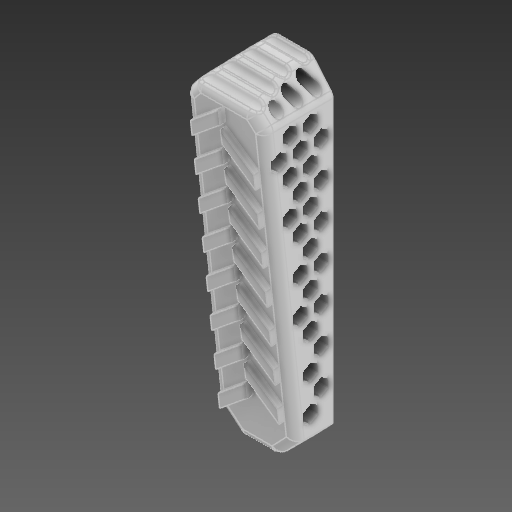
# Autodesk Inventor part: StockBack
Saved by Autodesk Inventor 2020.4 (Build 244396010, 396A)
## iProperties
Created: 2022-09-17
Part Number: StockBack
Material: Generic
Document SubType Name: Modeling
Designer: Val
Density: 1 g/cm^3
Appearance: Default
Author: Val
Autodesk Inventor part; units mm, degrees
ref_plane "Work Plane1" through (-11.1125, 103.225, 25.0771) normal (0, 0, -1) x (-1, 0, 0)
ref_plane "Work Plane2" through (-8.3683, 113.0409, 21.1281) normal (0, -0.1094954, 0.9939873) x (1, 0, 0)
ref_plane "YZ Plane" through (0, 0, 0) normal (1, 0, 0) x (0, 1, 0)
sketch "Base" plane through (0, 0, 0) normal (0, 0, 1) x (1, 0, 0)
  line L0 (0, 119.9075) -> (0, 0) construction
  line L1 (6.6224, 0) -> (0, 0)
  line L2 (14.2875, 7.9536) -> (6.6224, 0)
  line L3 (14.2875, 110.8887) -> (14.2875, 7.9536)
  line L4 (6.6224, 119.9075) -> (14.2875, 110.8887)
  line L5 (0, 119.9075) -> (6.6224, 119.9075)
  line L6 (0, 119.9075) -> (0, 0) construction
  line L7 (0, 119.9075) -> (-6.6224, 119.9075)
  line L8 (-6.6224, 119.9075) -> (-14.2875, 110.8887)
  line L9 (-14.2875, 110.8887) -> (-14.2875, 7.9536)
  line L10 (-14.2875, 7.9536) -> (-6.6224, 0)
  line L11 (-6.6224, 0) -> (0, 0)
  dimension "d0" = 136.058
  dimension "d1" = 139.638
  dimension "d2" = 90
  dimension "d3" = 40.362
  dimension "d4" = 90
  dimension "d5" = 43.942
  dimension "d6" = 14.2875
  dimension "d7" = 28.575
  dimension "d8" = 119.9075
  dimension "d9" = 14.2875
  dimension "d10" = 4.7684
  dimension "d11" = 82.6993
  dimension "d12" = 0
  dimension "d13" = 82.6993
  dimension "d14" = 4.7684
  constraints: 24 end point, 3 parallel, 1 horizontal, 1 vertical
  measures "d0" angle of L2 L3
  measures "d1" angle of L3 L4
  measures "d2" angle of L3 L7
  measures "d3" angle of L3 L8
  measures "d4" angle of L3 L11
  measures "d5" angle of L3 L10
  measures "d6" distance between parallel lines of L0 L3
  measures "d7" distance between parallel lines of L3 L9
  measures "d8" distance between parallel lines of L1 L5
  measures "d9" distance from line of point (0, 0) L3
  measures "d10" distance from line of point (0, 0) L2
  measures "d11" distance from line of point (0, 0) L4
  measures "d12" distance from line of point (0, 0) L1
  measures "d13" distance from line of point (0, 0) L8
  measures "d14" distance from line of point (0, 0) L10
extrude "BaseFeature" add sketch "Base" along normal blind 25.4
sketch "StockShapeProfile" plane through (-14.2875, 7.9536, 0) normal (-1, 0, 0) x (0, 0, 1)
  line L0 (-123.6771, 148.6169) -> (-186.3503, 165.9719) projected
  line L1 (-123.6771, 148.6169) -> (25.4, 107.3356)
  line L2 (-123.6771, 148.6169) -> (25.4, 148.6169)
  line L3 (25.4, 107.3356) -> (25.4, 148.6169)
  line L4 (25.4, 102.9352) -> (25.4, 0) projected
  point P0 (0, -7.9536)
  constraints: 6 end point, 2 collinear, 1 horizontal, 1 perpendicular
extrude "StockShapeFeature" cut sketch "StockShapeProfile" against normal through all both and the other way through all
sketch "StockProfile" plane through (-14.2875, 7.9536, 0) normal (-1, 0, 0) x (0, 0, 1)
  line L0 (25.4, 107.3356) -> (25.4, 102.9352) projected
  line L1 (25.4, 107.3356) -> (12.7, -7.9536)
  line L2 (0, -7.9536) -> (25.4, -7.9536) projected
  line L3 (25.4, 0) -> (25.4, -7.9536) projected
  line L4 (12.7, -7.9536) -> (25.4, -7.9536)
  line L5 (25.4, -7.9536) -> (25.4, 107.3356)
  constraints: 6 end point, 1 horizontal, 1 midpoint, 1 perpendicular
extrude "StockProfieFeature" cut sketch "StockProfile" against normal through all
fillet "StockFilletsFeature" radius 3.175 18 edges at (-14.2875, 110.8887, 12.4576) (-8.5849, 117.5983, 17.0611) (8.5849, 117.5983, 17.0611) (-14.2875, 7.9536, 6.7881) (-14.2875, 59.4212, 19.2457) (-12.4175, 113.089, 25.1576) (0, 115.2892, 25.4) (-10.4549, 3.9768, 13.1381) (10.4549, 3.9768, 13.1381) (14.2875, 59.4212, 19.2457) (14.2875, 110.8887, 12.4576) (12.4175, 113.089, 25.1576) (-6.6224, 119.9075, 4.3611) (6.6224, 119.9075, 4.3611) (3.3112, 119.9075, 8.7222) (-6.6224, 0, 6.35) (6.6224, 0, 6.35) (3.3112, 0, 12.7)
sketch "StockHoneycomb" plane through (-14.2875, 7.9536, 0) normal (-1, 0, 0) x (0, 0, 1)
  line L0 (7.9734, 94.5852) -> (5.2237, 96.1727)
  line L1 (5.2237, 96.1727) -> (5.2237, 99.3477)
  line L2 (5.2237, 99.3477) -> (7.9734, 100.9352)
  line L3 (7.9734, 100.9352) -> (10.723, 99.3477)
  line L4 (10.723, 99.3477) -> (10.723, 96.1727)
  line L5 (10.723, 96.1727) -> (7.9734, 94.5852)
  line L6 (0, 102.9352) -> (24.9153, 102.9352) projected
  line L7 (14.4726, 92.8531) -> (14.4726, 89.6781)
  line L8 (14.4726, 89.6781) -> (11.723, 88.0906)
  line L9 (11.723, 88.0906) -> (8.9734, 89.6781)
  line L10 (8.9734, 89.6781) -> (8.9734, 92.8531)
  line L11 (8.9734, 92.8531) -> (11.723, 94.4406)
  line L12 (11.723, 94.4406) -> (14.4726, 92.8531)
  line L13 (18.2222, 99.3477) -> (18.2222, 96.1727)
  line L14 (18.2222, 96.1727) -> (15.4726, 94.5852)
  line L15 (15.4726, 94.5852) -> (12.723, 96.1727)
  line L16 (12.723, 96.1727) -> (12.723, 99.3477)
  line L17 (12.723, 99.3477) -> (15.4726, 100.9352)
  line L18 (15.4726, 100.9352) -> (18.2222, 99.3477)
  line L19 (19.2222, 94.4406) -> (21.9719, 92.8531)
  line L20 (21.9719, 92.8531) -> (21.9719, 89.6781)
  line L21 (21.9719, 89.6781) -> (19.2222, 88.0906)
  line L22 (19.2222, 88.0906) -> (16.4726, 89.6781)
  line L23 (16.4726, 89.6781) -> (16.4726, 92.8531)
  line L24 (16.4726, 92.8531) -> (19.2222, 94.4406)
  line L25 (6.9734, 92.8531) -> (6.9734, 89.6781)
  line L26 (6.9734, 89.6781) -> (4.2237, 88.0906)
  line L27 (4.2237, 88.0906) -> (1.4741, 89.6781)
  line L28 (1.4741, 89.6781) -> (1.4741, 92.8531)
  line L29 (1.4741, 92.8531) -> (4.2237, 94.4406)
  line L30 (4.2237, 94.4406) -> (6.9734, 92.8531)
  line L31 (13.5761, 0) -> (24.9153, 102.9352) projected
  line L32 (10.723, 99.3477) -> (12.723, 99.3477) construction
  line L33 (4.2237, 91.2656) -> (19.2222, 91.2656) construction
  line L34 (7.9734, 87.9461) -> (5.2237, 86.3586)
  line L35 (5.2237, 86.3586) -> (5.2237, 83.1836)
  line L36 (5.2237, 83.1836) -> (7.9734, 81.5961)
  line L37 (7.9734, 81.5961) -> (10.723, 83.1836)
  line L38 (10.723, 83.1836) -> (10.723, 86.3586)
  line L39 (10.723, 86.3586) -> (7.9734, 87.9461)
  line L40 (18.2222, 83.1836) -> (18.2222, 86.3586)
  line L41 (18.2222, 86.3586) -> (15.4726, 87.9461)
  line L42 (15.4726, 87.9461) -> (12.723, 86.3586)
  line L43 (12.723, 86.3586) -> (12.723, 83.1836)
  line L44 (12.723, 83.1836) -> (15.4726, 81.5961)
  line L45 (15.4726, 81.5961) -> (18.2222, 83.1836)
  line L46 (5.2237, 84.7711) -> (18.2222, 84.7711) construction
  line L47 (14.4726, 76.689) -> (14.4726, 79.864)
  line L48 (14.4726, 79.864) -> (11.723, 81.4515)
  line L49 (11.723, 81.4515) -> (8.9734, 79.864)
  line L50 (8.9734, 79.864) -> (8.9734, 76.689)
  line L51 (8.9734, 76.689) -> (11.723, 75.1015)
  line L52 (11.723, 75.1015) -> (14.4726, 76.689)
  line L53 (19.2222, 75.1015) -> (21.9719, 76.689) construction
  line L54 (21.9719, 76.689) -> (21.9719, 79.864) construction
  line L55 (21.9719, 79.864) -> (19.2222, 81.4515) construction
  line L56 (19.2222, 81.4515) -> (16.4726, 79.864) construction
  line L57 (16.4726, 79.864) -> (16.4726, 76.689) construction
  line L58 (16.4726, 76.689) -> (19.2222, 75.1015) construction
  line L59 (6.9734, 76.689) -> (6.9734, 79.864)
  line L60 (6.9734, 79.864) -> (4.2237, 81.4515)
  line L61 (4.2237, 81.4515) -> (1.4741, 79.864)
  line L62 (1.4741, 79.864) -> (1.4741, 76.689)
  line L63 (1.4741, 76.689) -> (4.2237, 75.1015)
  line L64 (4.2237, 75.1015) -> (6.9734, 76.689)
  line L65 (4.2237, 78.2765) -> (19.2222, 78.2765) construction
  line L66 (5.2237, 70.1945) -> (5.2237, 73.3695)
  line L67 (5.2237, 73.3695) -> (7.9734, 74.957)
  line L68 (7.9734, 68.607) -> (5.2237, 70.1945)
  line L69 (10.723, 70.1945) -> (7.9734, 68.607)
  line L70 (10.723, 73.3695) -> (10.723, 70.1945)
  line L71 (7.9734, 74.957) -> (10.723, 73.3695)
  line L72 (12.723, 73.3695) -> (15.4726, 74.957)
  line L73 (15.4726, 74.957) -> (18.2222, 73.3695)
  line L74 (12.723, 70.1945) -> (12.723, 73.3695)
  line L75 (15.4726, 68.607) -> (12.723, 70.1945)
  line L76 (18.2222, 70.1945) -> (15.4726, 68.607)
  line L77 (18.2222, 73.3695) -> (18.2222, 70.1945)
  line L78 (0, 111.9539) -> (8.7222, 111.9539) construction
  line L79 (4.1309, 105.8244) -> (5.8691, 108.835) construction
  line L80 (5.8629, 104.8244) -> (7.6012, 107.835)
  line L81 (4.1371, 109.835) -> (2.3988, 106.8244)
  arc A0 (2.3988, 106.8244) -> (5.8629, 104.8244) centre (4.1309, 105.8244) ccw
  arc A1 (7.6012, 107.835) -> (4.1371, 109.835) centre (5.8691, 108.835) ccw
  line L82 (11.0591, 105.8244) -> (12.1387, 107.6942) construction
  line L83 (9.327, 106.8244) -> (10.4066, 108.6942)
  line L84 (13.8707, 106.6942) -> (12.7911, 104.8244)
  arc A2 (9.327, 106.8244) -> (12.7911, 104.8244) centre (11.0591, 105.8244) ccw
  arc A3 (13.8707, 106.6942) -> (10.4066, 108.6942) centre (12.1387, 107.6942) ccw
  line L85 (11.723, 68.4624) -> (14.4726, 66.8749)
  line L86 (14.4726, 66.8749) -> (14.4726, 63.6999)
  line L87 (14.4726, 63.6999) -> (11.723, 62.1124)
  line L88 (11.723, 62.1124) -> (8.9734, 63.6999)
  line L89 (8.9734, 63.6999) -> (8.9734, 66.8749)
  line L90 (8.9734, 66.8749) -> (11.723, 68.4624)
  line L91 (4.2237, 68.4624) -> (6.9734, 66.8749)
  line L92 (6.9734, 66.8749) -> (6.9734, 63.6999)
  line L93 (6.9734, 63.6999) -> (4.2237, 62.1124)
  line L94 (4.2237, 62.1124) -> (1.4741, 63.6999)
  line L95 (1.4741, 63.6999) -> (1.4741, 66.8749)
  line L96 (1.4741, 66.8749) -> (4.2237, 68.4624)
  line L97 (7.9734, 61.9679) -> (10.723, 60.3804)
  line L98 (10.723, 60.3804) -> (10.723, 57.2054)
  line L99 (10.723, 57.2054) -> (7.9734, 55.6179)
  line L100 (7.9734, 55.6179) -> (5.2237, 57.2054)
  line L101 (5.2237, 57.2054) -> (5.2237, 60.3804)
  line L102 (5.2237, 60.3804) -> (7.9734, 61.9679)
  line L103 (0, 110.835) -> (8.2907, 110.835) projected
  line L104 (21.5925, 103.8244) -> (0, 103.8244) projected
  line L105 (8.2907, 110.835) -> (21.9482, 107.0531) projected
  line L106 (0, 110.835) -> (0, 103.8244) projected
  line L107 (17.9873, 105.8244) -> (18.1119, 106.0402) construction
  line L108 (19.7193, 104.8244) -> (19.8439, 105.0402)
  line L109 (16.3798, 107.0402) -> (16.2552, 106.8244)
  arc A4 (16.2552, 106.8244) -> (19.7193, 104.8244) centre (17.9873, 105.8244) ccw
  arc A5 (19.8439, 105.0402) -> (16.3798, 107.0402) centre (18.1119, 106.0402) ccw
  point P0 (0, -7.9536)
  point P1 (7.9734, 97.7602)
  point P2 (11.723, 91.2656)
  point P3 (15.4726, 97.7602)
  point P4 (18.2222, 71.782)
  point P5 (5, 107.3297)
  point P6 (11.5989, 106.7593)
  point P7 (11.723, 65.2874)
  point P8 (4.2237, 65.2874)
  point P9 (7.9734, 58.7929)
  point P10 (18.0496, 105.9323)
  dimension "d21" = 3.175
  dimension "d22" = 2
  dimension "d24" = 2
  dimension "d25" = 2
  dimension "d26" = 2
  dimension "d27" = 2
  dimension "d28" = 2
  dimension "d29" = 2
  dimension "d30" = 2
  dimension "d31" = 1.4741
  dimension "d44" = 2
  dimension "d45" = 2
  dimension "d46" = 2
  dimension "d47" = 2
  dimension "d48" = 2
  dimension "d49" = 2
  dimension "d69" = 60
  dimension "d70" = 2
  dimension "d71" = 2
  dimension "d72" = 5
  dimension "d73" = 2
  constraints: 212 end point, 45 symmetric about line, 18 parallel, 18 tangent, 12 point on circle, 6 centre point, 5 midpoint, 2 equal radius, 1 horizontal, 104 other
  measures "d21" distance of L1.end L2.end
  measures "d22" distance from line of L6 L2.end
  measures "d24" distance between parallel lines of L5 L11
  measures "d25" distance between parallel lines of L15 L12
  measures "d26" distance between parallel lines of L4 L16
  measures "d27" distance between parallel lines of L24 L14
  measures "d28" distance between parallel lines of L30 L0
  measures "d29" distance between parallel lines of L10 L25
  measures "d30" distance between parallel lines of L23 L7
  measures "d31" distance from line of L31 L20.end
  measures "d44" distance from line of L75 L85.end
  measures "d45" distance between parallel lines of L90 L69
  measures "d46" distance between parallel lines of L68 L91
  measures "d47" distance between parallel lines of L89 L92
  measures "d48" distance between parallel lines of L93 L102
  measures "d49" distance between parallel lines of L88 L97
  measures "d69" angle of L78 L79
  measures "d70" radius of A1
  measures "d71" distance between parallel lines of L83 L80
  measures "d72" distance from line of L106 point (5, 107.33)
  measures "d73" distance between parallel lines of L84 L109
extrude "StockHoneycomb1Feature" cut sketch "StockHoneycomb" against normal through all contours L0 L1 L2 L3 L4 L5 | L7 L8 L9 L10 L11 L12 | L13 L14 L15 L16 L17 L18 | L19 L20 L21 L22 L23 L24 | L25 L26 L27 L28 L29 L30 | L39 L38 L37 L36 L35 L34 | L45 L44 L43 L42 L41 L40 | L52 L51 L50 L49 L48 L47 | L64 L63 L62 L61 L60 L59 | L66 L67 L71 L70 L69 L68 | L72 L73 L77 L76 L75 L74 | A0 L81 A1 L80 | A2 L83 A3 L84 | A4 L109 A5 L108 | L85 L86 L87 L88 L89 L90 | L91 L92 L93 L94 L95 L96 | L97 L98 L99 L100 L101 L102
sketch "StockHoneycomp2" plane through (14.2875, 7.9536, 0) normal (1, 0, 0) x (0, 0, -1)
  line L0 (-1.4741, 53.8858) -> (-1.4741, 50.7108)
  line L1 (-1.4741, 50.7108) -> (-4.2237, 49.1233)
  line L2 (-4.2237, 49.1233) -> (-6.9734, 50.7108)
  line L3 (-6.9734, 50.7108) -> (-6.9734, 53.8858)
  line L4 (-6.9734, 53.8858) -> (-4.2237, 55.4733)
  line L5 (-4.2237, 55.4733) -> (-1.4741, 53.8858)
  line L6 (-8.9734, 53.8858) -> (-8.9734, 50.7108)
  line L7 (-8.9734, 50.7108) -> (-11.723, 49.1233)
  line L8 (-11.723, 49.1233) -> (-14.4726, 50.7108)
  line L9 (-14.4726, 50.7108) -> (-14.4726, 53.8858)
  line L10 (-14.4726, 53.8858) -> (-11.723, 55.4733)
  line L11 (-11.723, 55.4733) -> (-8.9734, 53.8858)
  line L12 (-5.2237, 57.2054) -> (-7.9734, 55.6179) projected
  line L13 (-7.9734, 55.6179) -> (-10.723, 57.2054) projected
  line L14 (-8.9734, 53.8858) -> (-6.9734, 53.8858) construction
  line L15 (-7.9734, 48.9788) -> (-5.2237, 47.3913)
  line L16 (-5.2237, 47.3913) -> (-5.2237, 44.2163)
  line L17 (-5.2237, 44.2163) -> (-7.9734, 42.6288)
  line L18 (-7.9734, 42.6288) -> (-10.723, 44.2163)
  line L19 (-10.723, 44.2163) -> (-10.723, 47.3913)
  line L20 (-10.723, 47.3913) -> (-7.9734, 48.9788)
  line L21 (-4.2237, 42.4842) -> (-1.4741, 40.8967)
  line L22 (-1.4741, 40.8967) -> (-1.4741, 37.7217)
  line L23 (-1.4741, 37.7217) -> (-4.2237, 36.1342)
  line L24 (-4.2237, 36.1342) -> (-6.9734, 37.7217)
  line L25 (-6.9734, 37.7217) -> (-6.9734, 40.8967)
  line L26 (-6.9734, 40.8967) -> (-4.2237, 42.4842)
  line L27 (-8.9734, 40.8967) -> (-8.9734, 37.7217)
  line L28 (-8.9734, 37.7217) -> (-11.723, 36.1342)
  line L29 (-11.723, 36.1342) -> (-14.4726, 37.7217)
  line L30 (-14.4726, 37.7217) -> (-14.4726, 40.8967)
  line L31 (-14.4726, 40.8967) -> (-11.723, 42.4842)
  line L32 (-11.723, 42.4842) -> (-8.9734, 40.8967)
  line L33 (-8.9734, 40.8967) -> (-6.9734, 40.8967) construction
  line L34 (-7.9734, 35.9897) -> (-5.2237, 34.4022)
  line L35 (-5.2237, 34.4022) -> (-5.2237, 31.2272)
  line L36 (-5.2237, 31.2272) -> (-7.9734, 29.6397)
  line L37 (-7.9734, 29.6397) -> (-10.723, 31.2272)
  line L38 (-10.723, 31.2272) -> (-10.723, 34.4022)
  line L39 (-10.723, 34.4022) -> (-7.9734, 35.9897)
  line L40 (-4.2237, 29.4951) -> (-1.4741, 27.9076)
  line L41 (-1.4741, 27.9076) -> (-1.4741, 24.7326)
  line L42 (-1.4741, 24.7326) -> (-4.2237, 23.1451)
  line L43 (-4.2237, 23.1451) -> (-6.9734, 24.7326)
  line L44 (-6.9734, 24.7326) -> (-6.9734, 27.9076)
  line L45 (-6.9734, 27.9076) -> (-4.2237, 29.4951)
  line L46 (-10.723, 21.4131) -> (-7.9734, 23.0006)
  line L47 (-7.9734, 23.0006) -> (-5.2237, 21.4131)
  line L48 (-5.2237, 21.4131) -> (-5.2237, 18.2381)
  line L49 (-5.2237, 18.2381) -> (-7.9734, 16.6506)
  line L50 (-7.9734, 16.6506) -> (-10.723, 18.2381)
  line L51 (-10.723, 18.2381) -> (-10.723, 21.4131)
  line L52 (-7.9734, 29.6397) -> (-7.9734, 23.0006) construction
  line L53 (-4.2237, 16.506) -> (-1.4741, 14.9185)
  line L54 (-1.4741, 14.9185) -> (-1.4741, 11.7435)
  line L55 (-1.4741, 11.7435) -> (-4.2237, 10.156)
  line L56 (-4.2237, 10.156) -> (-6.9734, 11.7435)
  line L57 (-6.9734, 11.7435) -> (-6.9734, 14.9185)
  line L58 (-6.9734, 14.9185) -> (-4.2237, 16.506)
  line L59 (-4.2237, 23.1451) -> (-4.2237, 16.506) construction
  line L60 (-5.2237, 8.424) -> (-5.2237, 5.249)
  line L61 (-5.2237, 5.249) -> (-7.9734, 3.6615)
  line L62 (-7.9734, 3.6615) -> (-10.723, 5.249)
  line L63 (-10.723, 5.249) -> (-10.723, 8.424)
  line L64 (-10.723, 8.424) -> (-7.9734, 10.0115)
  line L65 (-7.9734, 10.0115) -> (-5.2237, 8.424)
  line L66 (-7.9734, 16.6506) -> (-7.9734, 10.0115) construction
  point P0 (0, -7.9536)
  point P1 (-4.2237, 52.2983)
  point P2 (-11.723, 52.2983)
  point P3 (-7.9734, 45.8038)
  point P4 (-4.2237, 39.3092)
  point P5 (-11.723, 39.3092)
  point P6 (-7.9734, 32.8147)
  point P7 (-4.2237, 26.3201)
  point P8 (-7.9734, 19.8256)
  point P9 (-4.2237, 13.331)
  point P10 (-7.9734, 6.8365)
  dimension "d52" = 2
  dimension "d53" = 2
  dimension "d54" = 2
  dimension "d55" = 2
  dimension "d56" = 2
  dimension "d57" = 2
  dimension "d58" = 2
  dimension "d59" = 2
  dimension "d60" = 2
  dimension "d61" = 2
  dimension "d62" = 2
  dimension "d63" = 2
  dimension "d64" = 1
  dimension "d65" = 2
  dimension "d66" = 2
  constraints: 130 end point, 22 parallel, 1 horizontal, 1 perpendicular, 1 vertical, 130 other
  measures "d52" distance between parallel lines of L12 L4
  measures "d53" distance between parallel lines of L13 L11
  measures "d54" distance between parallel lines of L3 L6
  measures "d55" distance between parallel lines of L7 L20
  measures "d56" distance between parallel lines of L2 L15
  measures "d57" distance between parallel lines of L17 L26
  measures "d58" distance between parallel lines of L18 L32
  measures "d59" distance between parallel lines of L25 L27
  measures "d60" distance between parallel lines of L24 L34
  measures "d61" distance between parallel lines of L28 L39
  measures "d62" distance between parallel lines of L45 L36
  measures "d63" distance between parallel lines of L43 L47
  measures "d64" distance between parallel lines of L52 L44
  measures "d65" distance between parallel lines of L49 L58
  measures "d66" distance between parallel lines of L56 L65
extrude "StockHoneycomb2Feature" cut sketch "StockHoneycomp2" against normal through all
sketch "Sketch5" plane through (-10.5475, 115.2892, 25.4) normal (0, -0.1094954, 0.9939873) x (1, 0, 0)
  line L0 (-3.74, -107.9849) -> (-3.74, -4.427) construction
  line L1 (3.9251, -115.9866) -> (-3.74, -107.9849) construction
  line L2 (17.1699, -115.9866) -> (3.9251, -115.9866) construction
  line L3 (24.835, -107.9849) -> (17.1699, -115.9866) construction
  line L4 (-0.565, -12.027) -> (10.5475, -2.7025)
  line L5 (-0.565, -12.027) -> (-0.565, -17.027)
  line L6 (-0.565, -17.027) -> (10.5475, -7.7025)
  line L7 (10.5475, -7.7025) -> (10.5475, -2.7025)
  line L8 (-3.74, -107.9849) -> (-3.74, -4.427) construction
  line L9 (2.1792, -2.7025) -> (18.9158, -2.7025) projected
  line L10 (-0.565, -5.9508) -> (2.1792, -2.7025) projected
  line L11 (-0.565, -107.046) -> (-0.565, -5.9508) construction
  line L12 (18.9158, -2.7025) -> (21.66, -5.9508) projected
  line L13 (21.66, -5.9508) -> (21.66, -107.046) construction
  line L14 (-2.1343, -3.1181) -> (23.2294, -3.1181) projected
  line L15 (10.5475, -3.1181) -> (10.5475, -117.3772) construction
  line L16 (10.5475, -9.2025) -> (10.5475, -14.2025)
  line L17 (10.5475, -9.2025) -> (21.66, -18.527)
  line L18 (21.66, -18.527) -> (21.66, -23.527)
  line L19 (21.66, -23.527) -> (10.5475, -14.2025)
  line L20 (-0.565, -25.027) -> (10.5475, -15.7025)
  line L21 (-0.565, -30.027) -> (10.5475, -20.7025)
  line L22 (-0.565, -25.027) -> (-0.565, -30.027)
  line L23 (10.5475, -20.7025) -> (10.5475, -15.7025)
  line L24 (-0.565, -38.027) -> (10.5475, -28.7025)
  line L25 (-0.565, -43.027) -> (10.5475, -33.7025)
  line L26 (-0.565, -38.027) -> (-0.565, -43.027)
  line L27 (10.5475, -33.7025) -> (10.5475, -28.7025)
  line L28 (-0.565, -51.027) -> (10.5475, -41.7025)
  line L29 (-0.565, -56.027) -> (10.5475, -46.7025)
  line L30 (-0.565, -51.027) -> (-0.565, -56.027)
  line L31 (10.5475, -46.7025) -> (10.5475, -41.7025)
  line L32 (-0.565, -64.027) -> (10.5475, -54.7025)
  line L33 (-0.565, -69.027) -> (10.5475, -59.7025)
  line L34 (-0.565, -64.027) -> (-0.565, -69.027)
  line L35 (10.5475, -59.7025) -> (10.5475, -54.7025)
  line L36 (-0.565, -77.027) -> (10.5475, -67.7025)
  line L37 (-0.565, -82.027) -> (10.5475, -72.7025)
  line L38 (-0.565, -77.027) -> (-0.565, -82.027)
  line L39 (10.5475, -72.7025) -> (10.5475, -67.7025)
  line L40 (-0.565, -90.027) -> (10.5475, -80.7025)
  line L41 (-0.565, -95.027) -> (10.5475, -85.7025)
  line L42 (-0.565, -90.027) -> (-0.565, -95.027)
  line L43 (10.5475, -85.7025) -> (10.5475, -80.7025)
  line L44 (-0.565, -103.027) -> (10.5475, -93.7025)
  line L45 (-0.565, -108.027) -> (10.5475, -98.7025)
  line L46 (-0.565, -103.027) -> (-0.565, -108.027)
  line L47 (10.5475, -98.7025) -> (10.5475, -93.7025)
  line L48 (10.5475, -22.2025) -> (21.66, -31.527)
  line L49 (10.5475, -22.2025) -> (10.5475, -27.2025)
  line L50 (21.66, -36.527) -> (10.5475, -27.2025)
  line L51 (21.66, -31.527) -> (21.66, -36.527)
  line L52 (10.5475, -35.2025) -> (21.66, -44.527)
  line L53 (10.5475, -35.2025) -> (10.5475, -40.2025)
  line L54 (21.66, -49.527) -> (10.5475, -40.2025)
  line L55 (21.66, -44.527) -> (21.66, -49.527)
  line L56 (10.5475, -48.2025) -> (21.66, -57.527)
  line L57 (10.5475, -48.2025) -> (10.5475, -53.2025)
  line L58 (21.66, -62.527) -> (10.5475, -53.2025)
  line L59 (21.66, -57.527) -> (21.66, -62.527)
  line L60 (10.5475, -61.2025) -> (21.66, -70.527)
  line L61 (10.5475, -61.2025) -> (10.5475, -66.2025)
  line L62 (21.66, -75.527) -> (10.5475, -66.2025)
  line L63 (21.66, -70.527) -> (21.66, -75.527)
  line L64 (10.5475, -74.2025) -> (21.66, -83.527)
  line L65 (10.5475, -74.2025) -> (10.5475, -79.2025)
  line L66 (21.66, -88.527) -> (10.5475, -79.2025)
  line L67 (21.66, -83.527) -> (21.66, -88.527)
  line L68 (10.5475, -87.2025) -> (21.66, -96.527)
  line L69 (10.5475, -87.2025) -> (10.5475, -92.2025)
  line L70 (21.66, -101.527) -> (10.5475, -92.2025)
  line L71 (21.66, -96.527) -> (21.66, -101.527)
  point P0 (10.5475, -3.1181)
  point P1 (10.0522, -3.1181)
  dimension "d42" = 5
  dimension "d74" = 50
  dimension "d75" = 50
  dimension "d76" = 1.5
  dimension "d79" = 13
  dimension "d84" = 1.5
  dimension "d87" = 13
  constraints: 122 end point, 6 vertical, 3 collinear, 3 equal length, 3 parallel, 2 midpoint, 104 other
  measures "d42" distance of L4.start L5.end
  measures "d74" angle of L11 L4
  measures "d75" angle of L13 L17
  measures "d76" distance of L6.end L16.start
  measures "d79" distance of L4.start L20.start
  measures "d84" distance of L20.end L16.end
  measures "d87" distance of L16.start L48.start
extrude "Extrusion6" add sketch "Sketch5" along normal blind 2 contours L4 L14 L7 L6 L5 | L17 L18 L19 L16 | L20 L23 L21 L22 | L24 L27 L25 L26 | L28 L31 L29 L30 | L32 L35 L33 L34 | L36 L39 L37 L38 | L40 L43 L41 L42 | L44 L47 L45 L46 | L48 L51 L50 L49 | L52 L55 L54 L53 | L56 L59 L58 L57 | L60 L63 L62 L61 | L64 L67 L66 L65 | L68 L71 L70 L69
sketch "Sketch7" plane through (-14.2875, 9.2345, 0) normal (-1, 0, 0) x (0, 0, 1)
  line L0 (22.7955, 106.7759) -> (9.138, 110.5578) construction
  circle A0 centre (10.3221, 111.0669) radius 2
  line L1 (8.2907, 110.673) -> (0, 110.673) construction
  line L2 (8.2907, 109.5541) -> (12.6724, 108.3408) construction
  circle A1 centre (2.7021, 111.5541) radius 2
  line L3 (0, 109.5541) -> (5.8691, 109.5541) construction
  circle A2 centre (16.422, 109.3777) radius 2
  line L4 (12.6724, 108.3408) -> (18.6456, 106.6867) construction
  circle A3 centre (22.522, 107.6886) radius 2
  line L5 (18.6456, 106.6867) -> (21.9482, 105.7722) construction
  line L6 (10.3221, 111.0669) -> (22.522, 107.6886) construction
  line L7 (2.7021, 111.5541) -> (10.3221, 111.0669) construction
  point P0 (0, -9.2345)
  dimension "d94" = 4
  dimension "d95" = 12.659
  dimension "d96" = 7.62
  dimension "d97" = 168.181
  constraints: 4 centre point, 4 end point, 4 tangent, 3 equal radius, 1 coincident, 1 midpoint
  measures "d94" diameter of A0
  measures "d95" distance of L6.start L6.end
  measures "d96" horizontal distance of L7.start L6.start
  measures "d97" angle of L0 L7
extrude "Extrusion7" cut sketch "Sketch7" against normal through all
fillet "Fillet2" radius 1 35 edges at (-10.8231, 114.9396, 22.2654) (-10.7876, 115.0066, 21.9491) (-10.7874, 115.0069, 21.9483) (-9.7165, 116.0322, 20.7313) (10.7876, 115.0067, 21.9482) (10.7876, 115.0066, 21.9491) (10.8231, 114.9396, 22.2654) (10.7874, 115.0069, 21.9483) (9.7165, 116.0322, 20.7313) (-9.7411, 115.2625, 23.6366) (-10.7875, 115.0068, 21.9492) (0, 115.4633, 23.889) (9.7412, 115.2625, 23.6366) (10.7875, 115.0068, 21.9492) (0, 116.6342, 20.5429) (8.2974, 117.7099, 14.6372) (8.9262, 116.943, 17.5236) (0, 118.3233, 14.443) (0, 117.3465, 17.9705) (-8.2974, 117.7099, 14.6372) (-8.9262, 116.943, 17.5236) (-7.4866, 118.6342, 11.4269) (-7.58, 118.7671, 9.0391) (-6.1005, 119.7613, 8.3964) (0, 119.9067, 8.3614) (6.1004, 119.7613, 8.3964) (7.58, 118.7671, 9.0391) (7.4866, 118.6342, 11.4269) (0, 119.0356, 11.8706) (-6.8584, 119.4112, 1.252) (-6.8585, 119.4112, 4.1521) (6.8585, 119.4112, 4.1521) (6.8584, 119.4112, 1.252) (0, 119.9075, 0.9067) (0, 119.9075, 4.4975)
sketch "MountHoles" plane through (0, 0, 0) normal (0, 0, -1) x (-1, 0, 0)
  circle A0 centre (6, 99.5875) radius 3 projected
  circle A1 centre (-6, 99.5875) radius 3 projected
  circle A2 centre (6, 20.32) radius 3 projected
  circle A3 centre (-6, 20.32) radius 3 projected
  point P0 (0, 0)
  dimension "d103" = 10
  dimension "d104" = 10
  dimension "d105" = 10
  dimension "d106" = 10
  constraints: 4 centre point, 4 coincident
equation "\"d84\" = d76"
equation "\"d103\" = d105"
equation "\"d104\" = d105"
equation "\"d106\" = d105"
body "Solid1"
